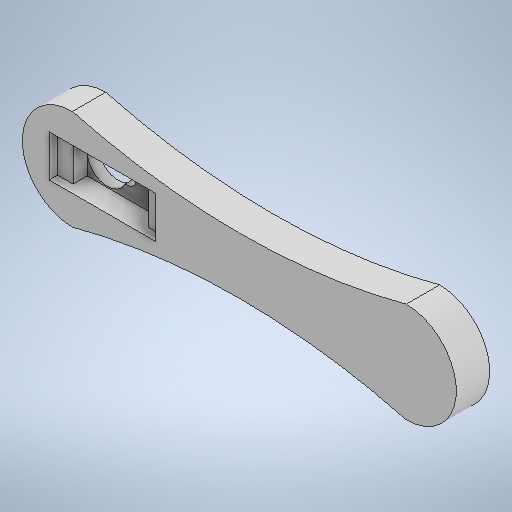
# Autodesk Inventor part: ramie gora
Saved by Autodesk Inventor 2025.2 (Build 292293000, 293)
## iProperties
Created: 2025-08-23
Part Number: ramie gora
Material: Ogólny
Document SubType Name: Modeling
Designer: IGOR
Density: 1 g/cm^3
Appearance: Domyślna
Author: IGOR
Autodesk Inventor part; units mm, degrees
ref_plane "YZ Plane" through (0, 0, 0) normal (1, 0, 0) x (0, 1, 0)
ref_plane "XZ Plane" through (0, 0, 0) normal (0, 1, 0) x (-1, 0, 0)
ref_plane "XY Plane" through (0, 0, 0) normal (0, 0, 1) x (1, 0, 0)
sketch "Szkic1" plane through (0, 0, 0) normal (0, 0, 1) x (1, 0, 0)
  line L0 (41.7431, -12.5229) -> (-50, 15) construction
  line L1 (-50, -15) -> (50, 15) construction
  arc A0 (-50, 15) -> (-50, -15) centre (-50, 0) ccw
  arc A1 (-50, 15) -> (50, 15) centre (0, 202.6168) ccw
  arc A2 (50, -15) -> (-50, -15) centre (0, -202.6168) ccw
  arc A3 (50, -15) -> (50, 15) centre (50, 0) ccw
  point P0 (0, 0)
  dimension "d4" = 194.165
  dimension "d5" = 194.165
  constraints: 8 point on circle, 4 centre point, 4 end point, 1 midpoint, 1 point on line
  measures "d4" radius of A1
  measures "d5" radius of A2
extrude "Wyciągnięcie proste1" add sketch "Szkic1" along normal blind 10
sketch "Szkic2" plane through (0, 0, 10) normal (0, 0, 1) x (1, 0, 0)
  line L0 (-25, -6.25) -> (-57, -6.25)
  line L1 (-57, -6.25) -> (-57, 6.25)
  line L2 (-57, 6.25) -> (-25, 6.25)
  line L3 (-25, 6.25) -> (-25, -6.25)
  line L4 (-25, -6.25) -> (-57, 6.25) construction
  line L5 (-57, -6.25) -> (-25, 6.25) construction
  point P0 (0, 0)
  point P1 (-41, 0)
  dimension "d9" = 32
  dimension "d10" = 12.5
  constraints: 12 end point, 2 midpoint, 2 parallel, 1 horizontal, 1 perpendicular
  measures "d9" distance of L1.end L2.end
  measures "d10" distance of L0.end L1.end
extrude "Wyciągnięcie proste2" cut sketch "Szkic2" against normal blind 2.5
sketch "Szkic3" plane through (0, 0, 7.5) normal (0, 0, 1) x (1, 0, 0)
  line L0 (-57, 6.25) -> (-25, 6.25) projected
  line L1 (-29.7, -6.25) -> (-52.3, -6.25)
  line L2 (-52.3, -6.25) -> (-52.3, 6.25)
  line L3 (-52.3, 6.25) -> (-29.7, 6.25)
  line L4 (-29.7, 6.25) -> (-29.7, -6.25)
  line L5 (-29.7, -6.25) -> (-52.3, 6.25) construction
  line L6 (-52.3, -6.25) -> (-29.7, 6.25) construction
  point P0 (0, 0)
  point P1 (-41, 0)
  dimension "d13" = 22.6
  constraints: 12 end point, 2 midpoint, 2 parallel, 1 horizontal, 1 perpendicular, 1 point on line
  measures "d13" distance of L2.end L3.end
extrude "Wyciągnięcie proste3" cut sketch "Szkic3" against normal blind 4.25
sketch "Szkic4" plane through (0, 0, 3.25) normal (0, 0, 1) x (1, 0, 0)
  arc A0 (-40.9075, 2.6308) -> (-40.9075, -2.6308) centre (-46.3, 0) ccw
  line L0 (-52.3, 6.25) -> (-52.3, -6.25)
  arc A1 (-40.9075, -2.6308) -> (-40.9075, 2.6308) centre (-40.3, 0) ccw
  point P0 (0, 0)
  dimension "d16" = 12
  dimension "d18" = 5.4
  constraints: 5 point on circle, 2 centre point, 2 end point, 1 vertical
  measures "d16" diameter of A0
  measures "d18" diameter of A1
extrude "Wyciągnięcie proste4" cut sketch "Szkic4" against normal blind 4.25
